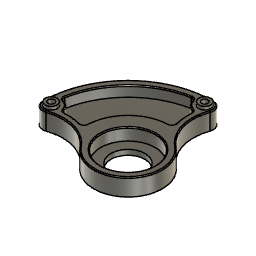
Tapa rodamiento (90°) v2 (Autodesk Fusion 360 design; units mm, degrees)
Autodesk Fusion 360 part; units mm, degrees
sketch "Boceto1" plane through (0, 0, 0) normal (0, 0, 1) x (1, 0, 0)
  circle A0 centre (-45, 0) radius 1.85
  circle A1 centre (0, 45) radius 1.85
  arc A2 (0, 50) -> (-50, 0) centre (0, 0) ccw
  arc A3 (-50, 0) -> (-43.3333, -4.714) centre (-45, 0) ccw
  arc A4 (-15.5556, -12.5708) -> (-43.3333, -4.714) centre (-35, -28.2843) ccw
  arc A5 (-15.5556, -12.5708) -> (12.5708, 15.5556) centre (0, 0) ccw
  arc A6 (4.714, 43.3333) -> (0, 50) centre (0, 45) ccw
  arc A7 (4.714, 43.3333) -> (12.5708, 15.5556) centre (28.2843, 35) ccw
  circle A8 centre (-45, 0) radius 3.5
  circle A9 centre (0, 45) radius 3.5
  circle A10 centre (0, 0) radius 16
  circle A11 centre (0, 0) radius 10
  dimension "d5" = 3.7
  dimension "d6" = 3.7
  dimension "d11" = 7
  dimension "d12" = 7
  dimension "d13" = 32
  dimension "d14" = 20
  constraint concentric A0 A8
  constraint concentric A6 A9
  constraint concentric A5 A11
  measures "d5" diameter of A0
  measures "d6" diameter of A1
  measures "d11" diameter of A8
  measures "d12" diameter of A9
  measures "d13" diameter of A10
  measures "d14" diameter of A11
extrude "Extruir1" add sketch "Boceto1" along normal blind 10 contours A2 A3 A4 A5 A6 A7 | A8 | A9 | A10
sketch "Boceto2" plane through (0, 0, 10) normal (0, 0, 1) x (-1, 0, 0)
  circle A0 centre (45, 0) radius 1.85
  circle A1 centre (0, -45) radius 1.85
  circle A2 centre (0, 0) radius 10
  arc A3 (0, -50) -> (50, 0) centre (0, 0) ccw
  arc A4 (50, 0) -> (43.3333, 4.714) centre (45, 0) ccw
  arc A5 (15.5556, 12.5708) -> (43.3333, 4.714) centre (35, 28.2843) ccw
  arc A6 (15.5556, 12.5708) -> (-12.5708, -15.5556) centre (0, 0) ccw
  arc A7 (-4.714, -43.3333) -> (-12.5708, -15.5556) centre (-28.2843, -35) ccw
  arc A8 (-4.714, -43.3333) -> (0, -50) centre (0, -45) ccw
  circle A9 centre (0, 0) radius 16
  circle A10 centre (0, -45) radius 3.5
  circle A11 centre (45, 0) radius 3.5
  dimension "d17" = 32
  dimension "d18" = 7
  dimension "d19" = 7
  constraint coincident A2.centre A3.centre
  constraint concentric A1 A10
  constraint concentric A0 A11
  measures "d17" diameter of A9
  measures "d18" diameter of A10
  measures "d19" diameter of A11
extrude "Extruir2" add sketch "Boceto2" along normal blind 1.82 contours A11
extrude "Extruir3" add sketch "Boceto2" along normal blind 1.82 contours A10
extrude "Extruir4" cut sketch "Boceto2" against normal blind 7 contours A9
sketch "Boceto3" plane through (0, 0, 10) normal (0, 0, 1) x (-1, 0, 0)
  circle A0 centre (0, 0) radius 16
  circle A1 centre (0, -45) radius 3.5
  circle A2 centre (45, 0) radius 3.5
  arc A3 (0, -50) -> (50, 0) centre (0, 0) ccw
  arc A4 (50, 0) -> (43.3333, 4.714) centre (45, 0) ccw
  arc A5 (15.5556, 12.5708) -> (43.3333, 4.714) centre (35, 28.2843) ccw
  arc A6 (15.5556, 12.5708) -> (-12.5708, -15.5556) centre (0, 0) ccw
  arc A7 (-4.714, -43.3333) -> (-12.5708, -15.5556) centre (-28.2843, -35) ccw
  arc A8 (-4.714, -43.3333) -> (0, -50) centre (0, -45) ccw
  arc A9 (39.2165, -1.5973) -> (43.725, -5.863) centre (45, 0) ccw
  arc A10 (27.502, 0.7883) -> (37.1386, -0.1354) centre (35, 28.2843) ccw
  arc A11 (1.0567, -24.9777) -> (24.9777, -1.0567) centre (0, 0) ccw
  arc A12 (0.1354, -37.1386) -> (-0.7883, -27.502) centre (-28.2843, -35) ccw
  arc A13 (5.863, -43.725) -> (1.5973, -39.2165) centre (0, -45) ccw
  arc A14 (8.1726, -45.2682) -> (45.2682, -8.1726) centre (0, 0) ccw
  arc A15 (5.863, -43.725) -> (8.1726, -45.2682) centre (7.8173, -43.3) ccw
  arc A16 (0.1354, -37.1386) -> (1.5973, -39.2165) centre (2.1297, -37.2887) ccw
  arc A17 (1.0567, -24.9777) -> (-0.7883, -27.502) centre (1.1413, -26.9759) ccw
  arc A18 (27.502, 0.7883) -> (24.9777, -1.0567) centre (26.9759, -1.1413) ccw
  arc A19 (39.2165, -1.5973) -> (37.1386, -0.1354) centre (37.2887, -2.1297) ccw
  arc A20 (45.2682, -8.1726) -> (43.725, -5.863) centre (43.3, -7.8173) ccw
  dimension "d32" = 2
  constraint coincident A0.centre A3.centre
  constraint tangent A13 A15
  constraint tangent A14 A15
  constraint tangent A12 A16
  constraint tangent A13 A16
  constraint equal A15 A16
  constraint tangent A11 A17
  constraint tangent A12 A17
  constraint equal A15 A17
  constraint tangent A10 A18
  constraint tangent A11 A18
  constraint equal A15 A18
  constraint tangent A9 A19
  constraint tangent A10 A19
  constraint equal A15 A19
  constraint tangent A9 A20
  constraint tangent A14 A20
  constraint equal A15 A20
  measures "d32" radius of A15
extrude "Extruir5" cut sketch "Boceto3" against normal blind 6 contours A9 A10 A11 A12 A13 A14 A15 A16 A17 A18 A19 A20
fillet "Empalme1" radius 0.5 6 edges at (-28.1959, -4.228, 10) (14.1421, -14.1421, 10) (4.228, 28.1959, 10) (4.0825, 47.8868, 10) (-35.3553, 35.3553, 10) (-47.8868, -4.0825, 10)
fillet "Empalme2" radius 0.5 12 edges at (-0.0857, 32.2808, 10) (0.4734, 25.7957, 10) (-17.6777, 17.6777, 10) (-25.7957, -0.4734, 10) (-32.2808, 0.0857, 10) (-38.4395, 0.494, 10) (-40.8763, 4.3584, 10) (-44.963, 6.7062, 10) (-32.5269, 32.5269, 10) (-6.7062, 44.963, 10) (-4.3584, 40.8763, 10) (-0.494, 38.4395, 10)
fillet "Empalme3" radius 0.5 1 edges at (14.9172, -5.7858, 10)
